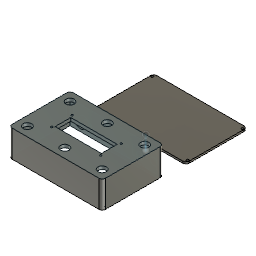
6SW_1602LCD_USBB_MIDI5PIN_DC (Autodesk Fusion 360 design; units mm, degrees)
Autodesk Fusion 360 part; units mm, degrees
note: some values were not read from the file. Set by a fixed rule: which sketch regions a step uses.
sketch "스케치1" plane through (0, 0, 0) normal (0, 0, 1) x (1, 0, 0)
  line L0 (72.5, -47.5) -> (-72.5, -47.5)
  line L1 (-72.5, -47.5) -> (-72.5, 47.5)
  line L2 (-72.5, 47.5) -> (72.5, 47.5)
  line L3 (72.5, 47.5) -> (72.5, -47.5)
  line L4 (72.5, -47.5) -> (-72.5, 47.5) construction
  line L5 (-72.5, -47.5) -> (72.5, 47.5) construction
  dimension "d1" = 145
  dimension "d2" = 95
  constraint horizontal L0
  constraint perpendicular L0 L1
  constraint parallel L0 L2
  constraint parallel L1 L3
  constraint coincident L4 origin
  constraint coincident L5 origin
  measures "d1" distance of L1.end L2.end
  measures "d2" distance of L0.end L1.end
extrude "돌출1" add sketch "스케치1" along normal blind 45 makes body 1
sketch "스케치2" plane through (0, 0, 0) normal (0, 0, -1) x (1, 0, 0)
  line L0 (-72.5, -47.5) -> (72.5, -47.5)
  line L1 (72.5, -47.5) -> (72.5, 47.5)
  line L2 (72.5, 47.5) -> (-72.5, 47.5)
  line L3 (-72.5, 47.5) -> (-72.5, -47.5)
  line L4 (67.5, -42.5) -> (-67.5, -42.5)
  line L5 (-67.5, -42.5) -> (-67.5, 42.5)
  line L6 (-67.5, 42.5) -> (67.5, 42.5)
  line L7 (67.5, 42.5) -> (67.5, -42.5)
  line L8 (67.5, -42.5) -> (-67.5, 42.5) construction
  line L9 (-67.5, -42.5) -> (67.5, 42.5) construction
  dimension "d5" = 135
  dimension "d6" = 85
  constraint horizontal L4
  constraint perpendicular L4 L5
  constraint parallel L4 L6
  constraint parallel L5 L7
  constraint coincident L8 origin
  constraint coincident L9 origin
  measures "d5" distance of L5.end L6.end
  measures "d6" distance of L4.end L5.end
extrude "돌출2" cut sketch "스케치2" against normal blind 40 contours L4 L5 L6 L7 bodies 1
sketch "스케치3" plane through (0, 0, 45) normal (0, 0, 1) x (-1, 0, 0)
sketch "스케치4" plane through (0, 0, 40) normal (0, 0, -1) x (1, 0, 0)
  line L0 (67.5, 42.5) -> (-67.5, 42.5)
  line L1 (-67.5, 42.5) -> (-67.5, -42.5)
  line L2 (-67.5, -42.5) -> (67.5, -42.5)
  line L3 (67.5, -42.5) -> (67.5, 42.5)
  circle A0 centre (55, -30) radius 6.5
  line L4 (67.5, 42.5) -> (55, 42.5)
  line L5 (55, 42.5) -> (55, 30)
  line L6 (55, 30) -> (67.5, 30)
  line L7 (67.5, 30) -> (67.5, 42.5)
  circle A1 centre (55, 30) radius 6.5
  line L8 (-67.5, 42.5) -> (-55, 42.5)
  line L9 (-55, 42.5) -> (-55, 30)
  line L10 (-55, 30) -> (-67.5, 30)
  line L11 (-67.5, 30) -> (-67.5, 42.5)
  circle A2 centre (-55, 30) radius 6.5
  line L12 (-67.5, -42.5) -> (-55, -42.5)
  line L13 (-55, -42.5) -> (-55, -30)
  line L14 (-55, -30) -> (-67.5, -30)
  line L15 (-67.5, -30) -> (-67.5, -42.5)
  circle A3 centre (-55, -30) radius 6.5
  line L16 (55, 30) -> (0, 30)
  circle A4 centre (0, 30) radius 6.5
  dimension "d9" = 13
  dimension "d10" = 12.5
  dimension "d11" = 12.5
  dimension "d12" = 13
  dimension "d13" = 12.5
  dimension "d14" = 12.5
  dimension "d15" = 13
  dimension "d16" = 12.5
  dimension "d17" = 12.5
  dimension "d18" = 13
  dimension "d19" = 13
  constraint horizontal L4
  constraint vertical L5
  constraint horizontal L6
  constraint vertical L7
  constraint coincident L0.start L3.end
  constraint coincident L5.end L6.start
  constraint horizontal L8
  constraint vertical L9
  constraint horizontal L10
  constraint vertical L11
  constraint coincident L0.end L1.start
  constraint coincident L9.end L10.start
  constraint horizontal L12
  constraint vertical L13
  constraint horizontal L14
  constraint vertical L15
  constraint coincident L1.end L2.start
  constraint coincident L13.end L14.start
  constraint perpendicular L5 L16
  constraint coincident L16.end A4.centre
  measures "d9" diameter of A0
  measures "d10" distance of L0.start L4.end
  measures "d11" distance of L0.start L6.end
  measures "d12" diameter of A1
  measures "d13" distance of L0.end L8.end
  measures "d14" distance of L0.end L10.end
  measures "d15" diameter of A2
  measures "d16" distance of L1.end L12.end
  measures "d17" distance of L1.end L14.end
  measures "d18" diameter of A3
  measures "d19" diameter of A4
extrude "돌출3" cut sketch "스케치4" against normal blind 40 contours L5 L6 A1 | L5 A1 L16 | L6 A1 L16 | L9 L10 A2 | L9 L10 A2 | L13 L14 A3 | L13 L14 A3 | A0 | A4 bodies 1
fillet "필렛1" radius 5 4 edges at (-72.5, -47.5, 22.5) (72.5, -47.5, 22.5) (72.5, 47.5, 22.5) (-72.5, 47.5, 22.5) on bodies 1
sketch "스케치5" plane through (0, 0, 40) normal (0, 0, -1) x (1, 0, 0)
  circle A0 centre (0, 30) radius 6.5
  circle A1 centre (55, 30) radius 6.5
  circle A2 centre (-55, 30) radius 6.5
  circle A3 centre (55, -30) radius 6.5
  circle A4 centre (-55, -30) radius 6.5
  line L0 (67.5, 42.5) -> (-67.5, 42.5)
  line L1 (-67.5, 42.5) -> (-67.5, -42.5)
  line L2 (-67.5, -42.5) -> (67.5, -42.5)
  line L3 (67.5, -42.5) -> (67.5, 42.5)
  circle A5 centre (38.0373, 15.4254) radius 1.5
  line L4 (36.0373, -12.2246) -> (-35.9627, -12.2246)
  line L5 (-35.9627, -12.2246) -> (-35.9627, 12.2754)
  line L6 (36.0373, 12.2754) -> (36.0373, -12.2246)
  line L7 (-35.9627, 12.2754) -> (36.0373, 12.2754)
  circle A6 centre (38.0373, -16.2546) radius 1.5
  circle A7 centre (-37.9627, -16.2546) radius 1.5
  circle A8 centre (-37.9627, 15.2754) radius 1.5
  line L8 (-36, 12.15) -> (36, 12.15)
  line L9 (36, 12.15) -> (36, -12.15)
  line L10 (36, -12.15) -> (-36, -12.15)
  line L11 (-36, -12.15) -> (-36, 12.15)
  line L12 (-36, 12.15) -> (36, -12.15) construction
  line L13 (36, 12.15) -> (-36, -12.15) construction
  dimension "d24" = 72
  constraint horizontal L8
  constraint perpendicular L8 L9
  constraint parallel L8 L10
  constraint parallel L9 L11
  constraint coincident L12 origin
  constraint coincident L13 origin
  measures "d24" distance of L9.end L10.end
extrude "돌출4" cut sketch "스케치5" against normal blind 40 contours A5 | L5 L8 L9 L10 | A6 | A7 | A8 bodies 1
sketch "스케치6" plane through (0, 47.5, 0) normal (0, 1, 0) x (-1, 0, 0)
  line L0 (67.5, 0) -> (67.5, 45)
  line L1 (67.5, 45) -> (-67.5, 45)
  line L2 (-67.5, 45) -> (-67.5, 0)
  line L3 (-67.5, 0) -> (67.5, 0)
  circle A0 centre (40.6045, 15.8083) radius 7.5
  circle A1 centre (51.6045, 15.8083) radius 1.25
  circle A2 centre (29.6045, 15.8083) radius 1.25
extrude "돌출5" cut sketch "스케치6" against normal blind 10 contours A0 | A1 | A2 bodies 1
sketch "스케치7" plane through (0, 47.5, 0) normal (0, 1, 0) x (-1, 0, 0)
  circle A0 centre (40.6045, 15.8083) radius 7.5
  circle A1 centre (51.6045, 15.8083) radius 1.25
  circle A2 centre (29.6045, 15.8083) radius 1.25
  line L0 (67.5, 0) -> (67.5, 45)
  line L1 (67.5, 45) -> (-67.5, 45)
  line L2 (-67.5, 45) -> (-67.5, 0)
  line L3 (-67.5, 0) -> (67.5, 0)
  circle A3 centre (-41.3409, 16.5935) radius 5.5
  dimension "d29" = 11
  measures "d29" diameter of A3
extrude "돌출6" cut sketch "스케치7" against normal blind 17 contours A3 bodies 1
sketch "스케치8" plane through (0, 47.5, 0) normal (0, 1, 0) x (-1, 0, 0)
  circle A0 centre (-41.3409, 16.5935) radius 5.5
  circle A1 centre (40.6045, 15.8083) radius 7.5
  circle A2 centre (51.6045, 15.8083) radius 1.25
  circle A3 centre (29.6045, 15.8083) radius 1.25
  line L0 (67.5, 0) -> (67.5, 45)
  line L1 (67.5, 45) -> (-67.5, 45)
  line L2 (-67.5, 45) -> (-67.5, 0)
  line L3 (-67.5, 0) -> (67.5, 0)
  line L4 (0, 15) -> (-15, 15)
  line L5 (-15, 15) -> (0, 15)
  line L6 (0, 15) -> (15, 15)
  circle A4 centre (-15, 15) radius 2
  circle A5 centre (15, 15) radius 2
  line L7 (7, 8) -> (-7, 8)
  line L8 (-7, 8) -> (-7, 22)
  line L9 (-7, 22) -> (7, 22)
  line L10 (7, 22) -> (7, 8)
  line L11 (7, 8) -> (-7, 22) construction
  line L12 (-7, 8) -> (7, 22) construction
  line L13 (0, 45) -> (0, 28)
  circle A6 centre (40.6045, 15.8083) radius 7.5
  circle A7 centre (29.6045, 15.8083) radius 1.25
  circle A8 centre (51.6045, 15.8083) radius 1.25
  circle A9 centre (40.6045, 33.8083) radius 7.5
  circle A10 centre (29.6045, 33.8083) radius 1.25
  circle A11 centre (51.6045, 33.8083) radius 1.25
  point P0 (0, 15)
  dimension "d32" = 15
  dimension "d33" = 15
  dimension "d34" = 4
  dimension "d35" = 4
  dimension "d36" = 14
  dimension "d37" = 14
  dimension "d39" = 17
  constraint horizontal L4
  constraint parallel L4 L6
  constraint coincident L4.end L5.start
  constraint coincident L6.end A5.centre
  constraint horizontal L7
  constraint perpendicular L7 L8
  constraint parallel L7 L9
  constraint parallel L8 L10
  constraint coincident L11 P0
  constraint coincident L12 P0
  constraint coincident P0 L4.start
  constraint midpoint L1 L13.start
  constraint perpendicular L1 L13
  measures "d32" distance of P0 L4.end
  measures "d33" distance of P0 L6.end
  measures "d34" diameter of A4
  measures "d35" diameter of A5
  measures "d36" distance of L8.end L9.end
  measures "d37" distance of L7.end L8.end
  measures "d39" distance of L13.start L13.end
sketch "스케치9" plane through (0, 42.5, 0) normal (0, -1, 0) x (1, 0, 0)
  circle A0 centre (41.3409, 16.5935) radius 5.5
  circle A1 centre (-40.6045, 15.8083) radius 7.5
  circle A2 centre (-51.6045, 15.8083) radius 1.25
  circle A3 centre (-29.6045, 15.8083) radius 1.25
  line L0 (-67.5, 0) -> (67.5, 0)
  line L1 (67.5, 0) -> (67.5, 40)
  line L2 (67.5, 40) -> (-67.5, 40)
  line L3 (-67.5, 40) -> (-67.5, 0)
  line L4 (50, 40) -> (50, 28)
  dimension "d38" = 12
  constraint coincident L2 L4.start
  constraint perpendicular L2 L4
  measures "d38" distance of L4.start L4.end
extrude "돌출7" add sketch "스케치8" against normal blind 5 contours A0 | A1 A6 | A2 A8 | A3 A7 bodies 1
sketch "스케치10" plane through (0, 47.5, 0) normal (0, 1, 0) x (-1, 0, 0)
  line L0 (67.5, 0) -> (67.5, 45)
  line L1 (67.5, 45) -> (-67.5, 45)
  line L2 (-67.5, 45) -> (-67.5, 0)
  line L3 (-67.5, 0) -> (67.5, 0)
  circle A0 centre (51.2975, 14.4272) radius 7.5
  circle A1 centre (40.2975, 14.4272) radius 1.25
  circle A2 centre (62.2975, 14.4272) radius 1.25
  line L4 (-38.277, 22) -> (-24.277, 22)
  line L5 (-38.277, 8) -> (-38.277, 22)
  line L6 (-24.277, 8) -> (-38.277, 8)
  line L7 (-24.277, 22) -> (-24.277, 8)
  circle A3 centre (-16.277, 15) radius 2
  circle A4 centre (-46.277, 15) radius 2
  circle A5 centre (-57.5124, 14.9346) radius 5.5
  line L8 (0, 45) -> (0, 28)
  line L9 (0, 28) -> (1.5663, 28)
  line L10 (1.5663, 28) -> (67.5, 28)
  line L11 (0, 28) -> (-66.6014, 28)
  dimension "d42" = 4
  dimension "d43" = 4
  dimension "d44" = 14
  dimension "d45" = 14
  dimension "d46" = 17
  constraint horizontal L6
  constraint perpendicular L5 L6
  constraint parallel L4 L6
  constraint parallel L5 L7
  constraint midpoint L1 L8.start
  constraint perpendicular L1 L8
  constraint perpendicular L8 L9
  constraint coincident L0 L10.end
  constraint perpendicular L0 L10
  constraint perpendicular L8 L11
  measures "d42" diameter of A4
  measures "d43" diameter of A3
  measures "d44" distance of L4.start L4.end
  measures "d45" distance of L5.start L4.start
  measures "d46" distance of L8.start L8.end
extrude "돌출8" cut sketch "스케치10" against normal blind 40 contours A0 | A1 | A2 | L4 L5 L6 L7 | A3 | A4 | A5 bodies 1
sketch "스케치11" plane through (72.5, 0, 0) normal (1, 0, 0) x (0, 1, 0)
  line L0 (42.5, 0) -> (42.5, 45)
  line L1 (42.5, 45) -> (-42.5, 45)
  line L2 (-42.5, 45) -> (-42.5, 0)
  line L3 (-42.5, 0) -> (42.5, 0)
sketch "스케치12" plane through (0, 0, 0) normal (0, 0, -1) x (1, 0, 0)
  line L0 (-67.5, -42.5) -> (-67.5, 42.5)
  line L1 (-67.5, 42.5) -> (67.5, 42.5)
  line L2 (67.5, 42.5) -> (67.5, -42.5)
  line L3 (67.5, -42.5) -> (-67.5, -42.5)
  arc A0 (-72.5, -42.5) -> (-67.5, -47.5) centre (-67.5, -42.5) ccw
  line L4 (-67.5, -47.5) -> (67.5, -47.5)
  arc A1 (67.5, -47.5) -> (72.5, -42.5) centre (67.5, -42.5) ccw
  line L5 (72.5, -42.5) -> (72.5, 42.5)
  arc A2 (72.5, 42.5) -> (67.5, 47.5) centre (67.5, 42.5) ccw
  line L6 (67.5, 47.5) -> (-67.5, 47.5)
  arc A3 (-67.5, 47.5) -> (-72.5, 42.5) centre (-67.5, 42.5) ccw
  line L7 (-72.5, 42.5) -> (-72.5, -42.5)
  line L8 (-72.5, 47.5) -> (72.5, -47.5) construction
  line L9 (72.5, 47.5) -> (-72.5, -47.5) construction
  line L10 (-72.5, 47.5) -> (-70, 47.5)
  line L11 (-70, 47.5) -> (-70, 42.5)
  line L12 (-70, 42.5) -> (-72.5, 42.5)
  line L13 (-72.5, 42.5) -> (-72.5, 47.5)
  circle A4 centre (-70, 42.5) radius 1.7
  line L14 (-72.5, -47.5) -> (-70, -47.5)
  line L15 (-70, -47.5) -> (-70, -42.5)
  line L16 (-70, -42.5) -> (-72.5, -42.5)
  line L17 (-72.5, -42.5) -> (-72.5, -47.5)
  circle A5 centre (-70, -42.5) radius 1.7
  dimension "d49" = 145
  dimension "d64" = 2.5
  dimension "d65" = 3.4
  dimension "d66" = 2.5
  dimension "d67" = 3.4
  constraint coincident L8 origin
  constraint coincident L9 origin
  constraint horizontal L10
  constraint vertical L11
  constraint horizontal L12
  constraint vertical L13
  constraint coincident L11.end L12.start
  constraint horizontal L14
  constraint vertical L15
  constraint horizontal L16
  constraint vertical L17
  constraint coincident L15.end L16.start
  measures "d49" distance of L8.end L9.end
  measures "d64" distance of L8.start L10.end
  measures "d65" diameter of A4
  measures "d66" distance of L9.end L14.end
  measures "d67" diameter of A5
sketch "스케치13" plane through (0, 0, 0) normal (1, 0, 0) x (0, 1, 0)
sketch "스케치14" plane through (0, 0, 0) normal (0, 0, 1) x (1, 0, 0)
  line L0 (72.5, 177.5) -> (-72.5, 177.5)
  line L1 (-72.5, 177.5) -> (-72.5, 82.5)
  line L2 (-72.5, 82.5) -> (72.5, 82.5)
  line L3 (72.5, 82.5) -> (72.5, 177.5)
  line L4 (72.5, 177.5) -> (-72.5, 82.5) construction
  line L5 (-72.5, 177.5) -> (72.5, 82.5) construction
  point P0 (0, 130)
  dimension "d50" = 145
  dimension "d51" = 95
  constraint horizontal L0
  constraint perpendicular L0 L1
  constraint parallel L0 L2
  constraint parallel L1 L3
  constraint coincident L4 P0
  constraint coincident L5 P0
  measures "d50" distance of L1.end L2.end
  measures "d51" distance of L0.end L1.end
extrude "돌출9" add sketch "스케치14" along normal blind 3 separate body makes body 2
fillet "필렛2" radius 5 4 edges at (72.5, 177.5, 1.5) (-72.5, 177.5, 1.5) (-72.5, 82.5, 1.5) (72.5, 82.5, 1.5) on bodies 2
sketch "스케치15" plane through (0, 0, 0) normal (0, 0, -1) x (1, 0, 0)
  line L0 (72.5, -47.5) -> (70, -47.5)
  line L1 (70, -47.5) -> (70, -42.5)
  line L2 (70, -42.5) -> (72.5, -42.5)
  line L3 (72.5, -42.5) -> (72.5, -47.5)
  circle A0 centre (70, -42.5) radius 1.7
  line L4 (72.5, 47.5) -> (70, 47.5)
  line L5 (70, 47.5) -> (70, 42.5)
  line L6 (70, 42.5) -> (72.5, 42.5)
  line L7 (72.5, 42.5) -> (72.5, 47.5)
  circle A1 centre (70, 42.5) radius 1.7
  line L8 (-67.5088, 42.4979) -> (-70.0088, 42.4979) construction
  dimension "d56" = 2.5
  dimension "d57" = 3.4
  dimension "d58" = 2.5
  dimension "d59" = 5
  dimension "d60" = 3.4
  dimension "d61" = 2.5
  constraint horizontal L0
  constraint vertical L1
  constraint horizontal L2
  constraint vertical L3
  constraint coincident L1.end L2.start
  constraint horizontal L4
  constraint vertical L5
  constraint horizontal L6
  constraint vertical L7
  constraint coincident L5.end L6.start
  constraint horizontal L8
  measures "d56" distance of L0.start L0.end
  measures "d57" diameter of A0
  measures "d58" distance of L4.start L4.end
  measures "d59" distance of L4.start L6.end
  measures "d60" diameter of A1
  measures "d61" distance of L8.start L8.end
extrude "돌출10" cut sketch "스케치15" against normal blind 7 contours L1 L2 A0 | L1 L2 A0 | L5 L6 A1 | L5 L6 A1 bodies 1
extrude "돌출11" cut sketch "스케치12" against normal blind 7 contours L15 L16 A5 | L15 L16 A5 | L11 L12 A4 | L11 L12 A4 bodies 1
sketch "스케치16" plane through (0, 0, 0) normal (0, 0, -1) x (1, 0, 0)
  arc A0 (72.5, -87.5) -> (67.5, -82.5) centre (67.5, -87.5) ccw
  line L0 (67.5, -82.5) -> (-67.5, -82.5)
  arc A1 (-67.5, -82.5) -> (-72.5, -87.5) centre (-67.5, -87.5) ccw
  line L1 (-72.5, -87.5) -> (-72.5, -172.5)
  arc A2 (-72.5, -172.5) -> (-67.5, -177.5) centre (-67.5, -172.5) ccw
  line L2 (-67.5, -177.5) -> (67.5, -177.5)
  arc A3 (67.5, -177.5) -> (72.5, -172.5) centre (67.5, -172.5) ccw
  line L3 (72.5, -172.5) -> (72.5, -87.5)
  line L4 (72.5, -172.5) -> (70, -172.5)
  circle A4 centre (70, -172.5) radius 1.7
  line L5 (72.5, -87.5) -> (70, -87.5)
  circle A5 centre (70, -87.5) radius 1.7
  line L6 (-72.5, -87.5) -> (-70, -87.5)
  circle A6 centre (-70, -87.5) radius 1.7
  line L7 (-72.5, -172.5) -> (-70, -172.5)
  circle A7 centre (-70, -172.5) radius 1.7
  dimension "d70" = 2.5
  dimension "d71" = 3.4
  dimension "d72" = 2.5
  dimension "d73" = 3.4
  dimension "d74" = 3.4
  dimension "d75" = 2.5
  dimension "d76" = 3.4
  constraint coincident A3.end L3.start
  constraint perpendicular L3 L4
  constraint coincident L4.end A4.centre
  constraint coincident A0.start L3.end
  constraint perpendicular L3 L5
  constraint coincident L5.end A5.centre
  constraint coincident A1.end L1.start
  constraint perpendicular L1 L6
  constraint coincident L6.end A6.centre
  constraint coincident L1.end A2.start
  constraint perpendicular L1 L7
  constraint coincident L7.end A7.centre
  measures "d70" distance of A3.end L4.end
  measures "d71" diameter of A4
  measures "d72" distance of A0.start L5.end
  measures "d73" diameter of A5
  measures "d74" diameter of A6
  measures "d75" distance of L1.end L7.end
  measures "d76" diameter of A7
extrude "돌출12" cut sketch "스케치16" against normal blind 40 contours A4 | A5 | A6 | A7 bodies 2
sketch "스케치17" plane through (0, 0, 40) normal (0, 0, -1) x (1, 0, 0)
  circle A0 centre (38.0373, 15.4254) radius 1.5
  circle A1 centre (38.0373, -16.2546) radius 1.5
  circle A2 centre (-37.9627, 15.2754) radius 1.5
  line L0 (-35.9627, 12.15) -> (36, 12.15)
  line L1 (36, 12.15) -> (36, -12.15)
  line L2 (36, -12.15) -> (-35.9627, -12.15)
  line L3 (-35.9627, -12.15) -> (-35.9627, 12.15)
  circle A3 centre (-37.9627, -16.2546) radius 1.5
  circle A4 centre (0, 30) radius 6.5
  circle A5 centre (55, 30) radius 6.5
  circle A6 centre (-55, 30) radius 6.5
  circle A7 centre (55, -30) radius 6.5
  circle A8 centre (-55, -30) radius 6.5
  line L4 (67.5, 42.5) -> (-67.5, 42.5)
  line L5 (-67.5, 42.5) -> (-67.5, -42.5)
  line L6 (-67.5, -42.5) -> (67.5, -42.5)
  line L7 (67.5, -42.5) -> (67.5, 42.5)
  circle A9 centre (0, -30) radius 6.5
  dimension "d79" = 13
  measures "d79" diameter of A9
extrude "돌출13" cut sketch "스케치17" against normal blind 15 contours A9 bodies 1
sketch "스케치18" plane through (0, 47.5, 0) normal (0, 1, 0) x (-1, 0, 0)
  line L0 (-38.277, 8) -> (-38.277, 22)
  line L1 (-38.277, 22) -> (-24.277, 22)
  line L2 (-24.277, 22) -> (-24.277, 8)
  line L3 (-24.277, 8) -> (-38.277, 8)
  circle A0 centre (62.2975, 14.4272) radius 1.25
  circle A1 centre (-16.277, 15) radius 2
  circle A2 centre (-57.5124, 14.9346) radius 5.5
  circle A3 centre (51.2975, 14.4272) radius 7.5
  circle A4 centre (40.2975, 14.4272) radius 1.25
  circle A5 centre (-46.277, 15) radius 2
  line L4 (67.5, 0) -> (67.5, 45)
  line L5 (67.5, 45) -> (-67.5, 45)
  line L6 (-67.5, 45) -> (-67.5, 0)
  line L7 (-67.5, 0) -> (67.5, 0)
  line L8 (-45, 45) -> (-45, 25)
  constraint coincident L5 L8.start
  constraint perpendicular L5 L8
extrude "돌출14" cut 1 faces at (22.5, -45.8333, 0) along direction (0, 0, 1) blind 3 on bodies 1 bodies 1
sketch "스케치19" plane through (-72.5, 0, 0) normal (-1, 0, 0) x (0, -1, 0)
  line L0 (-42.5, 3) -> (42.5, 3)
  line L1 (42.5, 3) -> (42.5, 45)
  line L2 (42.5, 45) -> (-42.5, 45)
  line L3 (-42.5, 45) -> (-42.5, 3)
sketch "스케치20" plane through (0, 0, 40) normal (0, 0, -1) x (1, 0, 0)
  circle A0 centre (0, -30) radius 6.5
  circle A1 centre (38.0373, 15.4254) radius 1.5
  circle A2 centre (38.0373, -16.2546) radius 1.5
  circle A3 centre (-37.9627, 15.2754) radius 1.5
  line L0 (-35.9627, 12.15) -> (36, 12.15)
  line L1 (36, 12.15) -> (36, -12.15)
  line L2 (36, -12.15) -> (-35.9627, -12.15)
  line L3 (-35.9627, -12.15) -> (-35.9627, 12.15)
  circle A4 centre (-37.9627, -16.2546) radius 1.5
  circle A5 centre (0, 30) radius 6.5
  circle A6 centre (55, 30) radius 6.5
  circle A7 centre (-55, 30) radius 6.5
  circle A8 centre (55, -30) radius 6.5
  circle A9 centre (-55, -30) radius 6.5
  line L4 (67.5, 42.5) -> (-67.5, 42.5)
  line L5 (-67.5, 42.5) -> (-67.5, -42.5)
  line L6 (-67.5, -42.5) -> (67.5, -42.5)
  line L7 (67.5, -42.5) -> (67.5, 42.5)
extrude "돌출15" add sketch "스케치20" against normal blind 5 contours A0 | A5 | A6 | A7 | A8 | A9 bodies 1
sketch "스케치21" plane through (0, 0, 40) normal (0, 0, -1) x (1, 0, 0)
  circle A0 centre (38.0373, 15.4254) radius 1.5
  circle A1 centre (38.0373, -16.2546) radius 1.5
  circle A2 centre (-37.9627, 15.2754) radius 1.5
  line L0 (-35.9627, 12.15) -> (36, 12.15)
  line L1 (36, 12.15) -> (36, -12.15)
  line L2 (36, -12.15) -> (-35.9627, -12.15)
  line L3 (-35.9627, -12.15) -> (-35.9627, 12.15)
  circle A3 centre (-37.9627, -16.2546) radius 1.5
  line L4 (67.5, 42.5) -> (-67.5, 42.5)
  line L5 (-67.5, 42.5) -> (-67.5, -42.5)
  line L6 (-67.5, -42.5) -> (67.5, -42.5)
  line L7 (67.5, -42.5) -> (67.5, 42.5)
  circle A4 centre (58, 33) radius 6.5
  circle A5 centre (58, -33) radius 6.5
  circle A6 centre (-58, -33) radius 6.5
  circle A7 centre (-58, 33) radius 6.5
  circle A8 centre (0, 33) radius 6.5
  circle A9 centre (0, -33) radius 6.5
  dimension "d86" = 13
  dimension "d87" = 13
  dimension "d88" = 13
  dimension "d89" = 13
  dimension "d90" = 13
  dimension "d91" = 13
  measures "d86" diameter of A4
  measures "d87" diameter of A5
  measures "d88" diameter of A6
  measures "d89" diameter of A7
  measures "d90" diameter of A8
  measures "d91" diameter of A9
extrude "돌출16" cut sketch "스케치21" against normal blind 30 contours A4 | A5 | A6 | A7 | A8 | A9 bodies 1
sketch "스케치22" plane through (0, 0, 45) normal (0, 0, 1) x (-1, 0, 0)
  circle A0 centre (0, 33) radius 6.5
  circle A1 centre (0, -33) radius 6.5
  circle A2 centre (58, -33) radius 6.5
  circle A3 centre (-58, 33) radius 6.5
  circle A4 centre (-58, -33) radius 6.5
  circle A5 centre (58, 33) radius 6.5
  circle A6 centre (-38.0373, 15.4254) radius 1.5
  circle A7 centre (-38.0373, -16.2546) radius 1.5
  circle A8 centre (37.9627, 15.2754) radius 1.5
  line L0 (-36, 12.15) -> (35.9627, 12.15)
  line L1 (35.9627, 12.15) -> (35.9627, -12.15)
  line L2 (35.9627, -12.15) -> (-36, -12.15)
  line L3 (-36, -12.15) -> (-36, 12.15)
  circle A9 centre (37.9627, -16.2546) radius 1.5
  arc A10 (67.5, -47.5) -> (72.5, -42.5) centre (67.5, -42.5) ccw
  line L4 (72.5, -42.5) -> (72.5, 42.5)
  arc A11 (72.5, 42.5) -> (67.5, 47.5) centre (67.5, 42.5) ccw
  line L5 (67.5, 47.5) -> (-67.5, 47.5)
  arc A12 (-67.5, 47.5) -> (-72.5, 42.5) centre (-67.5, 42.5) ccw
  line L6 (-72.5, 42.5) -> (-72.5, -42.5)
  arc A13 (-72.5, -42.5) -> (-67.5, -47.5) centre (-67.5, -42.5) ccw
  line L7 (-67.5, -47.5) -> (67.5, -47.5)
